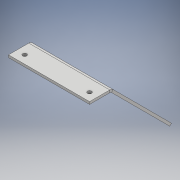
# Autodesk Inventor part: LRFマウント
Saved by Autodesk Inventor 2017 (Build 210142000, 142)
## iProperties
Part Number: LRFマウント
Material: 一般
Document SubType Name: Sheet Metal
Designer: highs
Density: 1 g/cm^3
Appearance: 既定
Sheet Metal Rule: Default_mm
Flat Pattern Width: 10 cm
Flat Pattern Length: 13 cm
Flat Pattern Area: 130 cm^2
Sheet Metal Width: 100.000 mm
Sheet Metal Length: 130.000 mm
Sheet Metal Area: 13000.000 mm^2
Author: highs
Autodesk Inventor part; units mm, degrees
ref_plane "YZ Plane" through (0, 0, 0) normal (1, 0, 0) x (0, 1, 0)
ref_plane "XZ Plane" through (0, 0, 0) normal (0, 1, 0) x (-1, 0, 0)
ref_plane "XY Plane" through (0, 0, 0) normal (0, 0, 1) x (1, 0, 0)
sketch "スケッチ1" plane through (0, 0, 0) normal (0, 0, 1) x (1, 0, 0)
  line L0 (0, 0) -> (100, 0)
  line L1 (100, 0) -> (100, 130)
  line L2 (100, 130) -> (0, 130)
  line L3 (0, 130) -> (0, 0)
  line L4 (0, 10) -> (100, 10) construction
  circle A0 centre (10, 10) radius 2.5
  circle A1 centre (90, 10) radius 2.5
  circle A2 centre (22, 100) radius 2
  circle A3 centre (22, 44) radius 2
  circle A4 centre (78, 100) radius 2
  circle A5 centre (78, 44) radius 2
  line L5 (50, 130) -> (50, 0) construction
  line L6 (0, 72) -> (100, 72) construction
  line L7 (22, 44) -> (78, 44) construction
  line L8 (78, 44) -> (78, 100) construction
  line L9 (78, 100) -> (22, 100) construction
  line L10 (22, 100) -> (22, 44) construction
  line L11 (22, 44) -> (78, 100) construction
  line L12 (78, 44) -> (22, 100) construction
  line L13 (0, 20) -> (100, 20) construction
  point P0 (50, 72)
  dimension "d0" = 5
  dimension "d1" = 10
  dimension "d2" = 10
  dimension "d3" = 10
  dimension "d4" = 100
  dimension "d5" = 130
  dimension "d12" = 4
  dimension "d21" = 56
  dimension "d22" = 56
  dimension "d25" = 20
  dimension "d27" = 30
  constraints: 28 end point, 8 point on line, 6 centre point, 5 midpoint, 5 perpendicular, 4 equal radius, 4 parallel, 2 coincident, 2 horizontal
  measures "d0" diameter of A0
  measures "d1" distance from line of L3 A0.centre
  measures "d2" distance between parallel lines of L0 L4
  measures "d3" distance from line of L1 A1.centre
  measures "d4" distance of L0.start L0.end
  measures "d5" distance of L2.end L0.start
  measures "d12" diameter of A2
  measures "d21" distance of L7.end L8.end
  measures "d22" distance of L8.end L9.end
  measures "d25" distance between parallel lines of L0 L13
  measures "d27" distance between parallel lines of L2 L9
extrude "押し出し1" add sketch "スケッチ1" along normal blind 3
sketch "スケッチ2" plane through (0, 0, 3) normal (0, 0, 1) x (1, 0, 0)
  line L0 (33, 150) -> (67, 150)
  line L1 (67, 150) -> (67, 110)
  line L2 (67, 110) -> (33, 110)
  line L3 (33, 110) -> (33, 150)
  line L4 (100, 130) -> (0, 130) projected
  line L5 (33, 150) -> (67, 110) construction
  line L6 (67, 150) -> (33, 110) construction
  point P0 (0, 0)
  point P1 (50, 130)
  dimension "d28" = 20
  dimension "d29" = 34
  constraints: 12 end point, 3 midpoint, 2 parallel, 1 horizontal, 1 perpendicular
  measures "d28" distance between parallel lines of L4 L2
  measures "d29" distance of L0.start L0.end
extrude "押し出し2" cut sketch "スケッチ2" against normal up to next
fillet "フィレット1" radius 1.5 2 edges at (67, 110, 1.5) (33, 110, 1.5)
sketch "スケッチ4" plane through (0, 0, 0) normal (0, 0, -1) x (-1, 0, 0)
  line L0 (-100, 0) -> (-100, 130) projected
  line L1 (-100, 25) -> (0, 25)
  line L2 (0, 130) -> (0, 0) projected
  line L3 (0, 25) -> (0, 0)
  line L4 (0, 0) -> (-100, 0)
  line L5 (-100, 0) -> (-100, 25)
  dimension "d40" = 25
  constraints: 8 end point, 3 perpendicular, 1 horizontal, 1 point on line
  measures "d40" distance between parallel lines of L4 L1
fold "折り曲げ1" angle 45 bend radius 3 thickness 3 k factor 0.44 line from (100, 25, 0) to (0, 25, 0) line at bend start moving side (0, 1, 0) folds toward (0, 0, -1)
equation "\"d34\" = BendReliefWidth"
equation "\"d35\" = BendReliefDepth"
equation "\"d36\" = MinimumRemnant"
equation "\"d37\" = BendRadius"
equation "\"d39\" = BendRadius"
equation "\"BendRadius\" = Thickness"
equation "\"BendReliefWidth\" = Thickness"
equation "\"BendReliefDepth\" = 0.5 * Thickness"
equation "\"CornerReliefSize\" = 4 * Thickness"
equation "\"MinimumRemnant\" = 2 * Thickness"
equation "\"TransitionRadius\" = BendRadius"
equation "\"JacobiRadiusSize\" = BendRadius"
equation "\"GapSize\" = Thickness"
equation "\"Thickness\" = 3"
